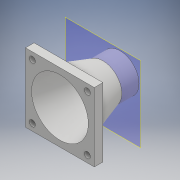
# Autodesk Inventor part: FanAdapter
Saved by Autodesk Inventor 2018 (Build 220112000, 112)
## iProperties
Created: 2018-11-08
Part Number: FanAdapter
Material: Generic
Document SubType Name: Modeling
Designer: reinert
Density: 1 g/cm^3
Appearance: Default
Author: reinert
Autodesk Inventor part; units mm, degrees
ref_plane "YZ Plane" through (0, 0, 0) normal (1, 0, 0) x (0, 1, 0)
ref_plane "XZ Plane" through (0, 0, 0) normal (0, 1, 0) x (-1, 0, 0)
ref_plane "XY Plane" through (0, 0, 0) normal (0, 0, 1) x (1, 0, 0)
sketch "Sketch1" plane through (0, 0, 0) normal (0, 1, 0) x (-1, 0, 0)
  line L0 (0, 0) -> (40, 0)
  line L1 (40, 0) -> (40, -40)
  line L2 (40, -40) -> (0, -40)
  line L3 (0, -40) -> (0, 0)
  dimension "d0" = 40
  dimension "d1" = 40
  constraints: 8 end point, 2 parallel, 1 horizontal, 1 perpendicular
  measures "d0" distance of L1.end L2.end
  measures "d1" distance of L0.end L1.end
extrude "Extrusion1" add sketch "Sketch1" along normal blind 5
sketch "Sketch2" plane through (0, 5, 0) normal (0, 1, 0) x (1, 0, 0)
  circle A0 centre (-20, 20) radius 17.5
  point P0 (0, 0)
  dimension "d4" = 35
  constraints: 1 centre point
  measures "d4" diameter of A0
ref_plane "Work Plane1" through (0, 25, 0) normal (0, 1, 0) x (1, 0, 0)
sketch "Sketch3" plane through (0, 25, 0) normal (0, 1, 0) x (1, 0, 0)
  circle A0 centre (-20, 20) radius 11
  point P0 (0, 0)
  dimension "d6" = 22
  constraints: 1 centre point
  measures "d6" diameter of A0
loft "Loft1" add profiles "Sketch2", "Sketch3"
sketch "Sketch6" plane through (0, 25, 0) normal (0, 1, 0) x (1, 0, 0)
  circle A0 centre (-20, 20) radius 9
  circle A1 centre (-20, 20) radius 11 projected
  point P0 (0, 0)
  dimension "d15" = 18
  constraints: 1 centre point, 1 concentric
  measures "d15" diameter of A0
sketch "Sketch8" plane through (0, 0, 0) normal (0, -1, 0) x (1, 0, 0)
  circle A0 centre (-20, -20) radius 16.5
  point P0 (0, 0)
  dimension "d16" = 33
  constraints: 1 centre point, 1 coincident
  measures "d16" diameter of A0
loft "Loft2" cut profiles "Sketch8", "Sketch6" contours all / A0
sketch "Sketch9" plane through (0, 25, 0) normal (0, 1, 0) x (1, 0, 0)
  circle A0 centre (-20, 20) radius 11
  circle A1 centre (-20, 20) radius 9
  point P0 (0, 0)
  dimension "d21" = 22
  dimension "d22" = 18
  constraints: 2 centre point, 1 coincident
  measures "d21" diameter of A0
  measures "d22" diameter of A1
extrude "Extrusion3" add sketch "Sketch9" along normal blind 10
hole "Hole1" at (-36, 5, -4) direction (0, -1, 0) diameter 3.5 end through all
hole "Hole2" at (-4, 5, -4) direction (0, -1, 0) diameter 3.5 end through all
hole "Hole3" at (-4, 5, -36) direction (0, -1, 0) diameter 3.5 end through all
hole "Hole4" at (-36, 5, -36) direction (0, -1, 0) diameter 3.5 end through all
body "Solid1"
